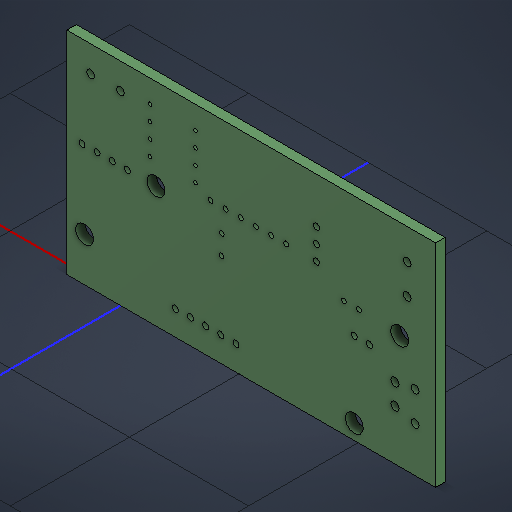
# Autodesk Inventor part: 000.006.001 - Плата
Saved by Autodesk Inventor 2025 (Build 290162000, 162)
## iProperties
Created: 2024-08-12
Part Number: 000.006.001 - Плата
Material: Типовые
Document SubType Name: Modeling
Designer: IvanPetrov
Density: 1 g/cm^3
Appearance: Контур панели
Author: IvanPetrov
Autodesk Inventor part; units mm, degrees
ref_plane "YZ Plane" through (0, 0, 0) normal (1, 0, 0) x (0, 1, 0)
ref_plane "XZ Plane" through (0, 0, 0) normal (0, 1, 0) x (-1, 0, 0)
ref_plane "XY Plane" through (0, 0, 0) normal (0, 0, 1) x (1, 0, 0)
sketch "Эскиз1" plane through (0, 0, 0) normal (0, 0, 1) x (1, 0, 0)
  line L0 (-8.89, 0) -> (53.01, 0)
  line L1 (53.01, 0) -> (53.01, 35.55)
  line L2 (53.01, 35.55) -> (-8.89, 35.55)
  line L3 (-8.89, 35.55) -> (-8.89, 0)
  circle A0 centre (15.24, 22.86) radius 0.405
  circle A1 centre (17.78, 22.86) radius 0.405
  circle A2 centre (20.32, 22.86) radius 0.405
  circle A3 centre (22.86, 22.86) radius 0.405
  circle A4 centre (25.4, 22.86) radius 0.405
  circle A5 centre (27.94, 22.86) radius 0.405
  circle A6 centre (37.62, 19.41) radius 0.405
  circle A7 centre (40.16, 19.41) radius 0.405
  circle A8 centre (0.1, 31.17) radius 0.65
  circle A9 centre (-4.9, 31.17) radius 0.65
  circle A10 centre (1.27, 20.32) radius 0.51
  circle A11 centre (-1.27, 20.32) radius 0.51
  circle A12 centre (-3.81, 20.32) radius 0.51
  circle A13 centre (-6.35, 20.32) radius 0.51
  circle A14 centre (48.26, 25.4) radius 0.65
  circle A15 centre (48.26, 30.4) radius 0.65
  circle A16 centre (9.33, 4.16) radius 0.51
  circle A17 centre (11.87, 4.16) radius 0.51
  circle A18 centre (14.41, 4.16) radius 0.51
  circle A19 centre (16.95, 4.16) radius 0.51
  circle A20 centre (19.49, 4.16) radius 0.51
  circle A21 centre (39.37, 15.24) radius 0.51
  circle A22 centre (41.91, 15.24) radius 0.51
  circle A23 centre (49.59, 7.57) radius 0.65
  circle A24 centre (49.59, 12.57) radius 0.65
  circle A25 centre (46.2, 8.43) radius 0.7
  circle A26 centre (46.2, 11.93) radius 0.7
  circle A27 centre (12.7, 24.13) radius 0.3
  circle A28 centre (5.08, 26.67) radius 0.3
  circle A29 centre (5.08, 24.13) radius 0.3
  circle A30 centre (12.7, 26.67) radius 0.3
  circle A31 centre (5.08, 31.75) radius 0.3
  circle A32 centre (5.08, 29.21) radius 0.3
  circle A33 centre (12.7, 29.21) radius 0.3
  circle A34 centre (12.7, 31.75) radius 0.3
  circle A35 centre (33.02, 25.4) radius 0.5
  circle A36 centre (33.02, 27.94) radius 0.5
  circle A37 centre (33.02, 22.86) radius 0.5
  circle A38 centre (-5.9225, 7.3465) radius 1.5
  circle A39 centre (39.37, 2.54) radius 1.5
  circle A40 centre (46.99, 19.05) radius 1.5
  circle A41 centre (6.0563, 20.3433) radius 1.5
  circle A42 centre (17.1236, 18.9948) radius 0.4
  circle A43 centre (17.0778, 15.6995) radius 0.4
  constraints: 44 centre point, 8 end point
extrude "OmniBot_motor_driver.brdКонтур" add sketch "Эскиз1" along normal blind 1.6
